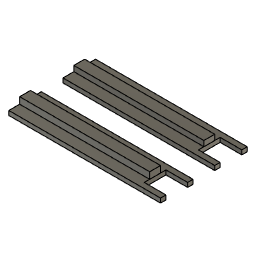
Abdeckung Profielschiene oben (Autodesk Fusion 360 design; units mm, degrees)
Autodesk Fusion 360 part; units mm, degrees
sketch "Skizze1" plane through (0, 0, 0) normal (0, 0, 1) x (1, 0, 0)
  line L0 (0, 0) -> (280, 0)
  line L1 (280, 0) -> (280, 30)
  line L2 (280, 30) -> (0, 30)
  line L3 (0, 30) -> (0, 0)
  dimension "d1" = 30
  dimension "d2" = 280
  constraint horizontal L0
  constraint vertical L1
  constraint horizontal L2
  constraint vertical L3
  constraint coincident L0.start L3.end
  measures "d1" distance of L0.start L2.end
  measures "d2" distance of L0.start L0.end
extrude "Extrusion1" add sketch "Skizze1" along normal blind 1 makes body 1
sketch "Skizze2" plane through (0, 0, 1) normal (0, 0, 1) x (-1, 0, 0)
  line L0 (0, -30) -> (0, 0)
  line L1 (0, 0) -> (-280, 0)
  line L2 (-280, 0) -> (-280, -30)
  line L3 (-280, -30) -> (0, -30)
  line L4 (0, -25) -> (-20, -25)
  line L5 (-20, -25) -> (-20, -5)
  line L6 (-20, -5) -> (0, -5)
  line L7 (0, -5) -> (0, -25)
  line L8 (-280, -25) -> (-260, -25)
  line L9 (-260, -25) -> (-260, -5)
  line L10 (-260, -5) -> (-280, -5)
  line L11 (-280, -5) -> (-280, -25)
  dimension "d5" = 20
  dimension "d6" = 20
  dimension "d7" = 5
  dimension "d8" = 5
  dimension "d9" = 20
  dimension "d10" = 20
  dimension "d11" = 5
  constraint horizontal L4
  constraint vertical L5
  constraint horizontal L6
  constraint vertical L7
  constraint coincident L0 L4.start
  constraint horizontal L8
  constraint vertical L9
  constraint horizontal L10
  constraint vertical L11
  constraint coincident L2 L8.start
  measures "d5" distance of L4.start L4.end
  measures "d6" distance of L4.start L6.end
  measures "d7" distance of L1 L6
  measures "d8" distance of L3 L4
  measures "d9" distance of L8.start L8.end
  measures "d10" distance of L8.start L10.end
  measures "d11" distance of L1 L10
extrude "Extrusion2" cut sketch "Skizze2" against normal blind 10 contours L0 L4 L5 L6 L7 | L2 L8 L9 L10 L11 bodies 1
sketch "Skizze3" plane through (0, 0, 1) normal (0, 0, 1) x (-1, 0, 0)
  line L0 (-260, -25) -> (-280, -25)
  line L1 (-280, -25) -> (-280, -30)
  line L2 (-280, -30) -> (0, -30)
  line L3 (0, -30) -> (0, -25)
  line L4 (0, -25) -> (-20, -25)
  line L5 (-20, -25) -> (-20, -5)
  line L6 (-20, -5) -> (0, -5)
  line L7 (0, -5) -> (0, 0)
  line L8 (0, 0) -> (-280, 0)
  line L9 (-280, 0) -> (-280, -5)
  line L10 (-280, -5) -> (-260, -5)
  line L11 (-260, -5) -> (-260, -25)
  line L12 (-259.9999, -20) -> (-20, -20)
  line L13 (-20, -20) -> (-20, -10)
  line L14 (-20, -10) -> (-259.9999, -10)
  line L15 (-259.9999, -10) -> (-259.9999, -20)
  dimension "d14" = 10
  dimension "d16" = 10
  constraint horizontal L12
  constraint vertical L13
  constraint horizontal L14
  constraint vertical L15
  measures "d14" distance of L8 L14
  measures "d16" distance of L2 L12
extrude "Extrusion3" add sketch "Skizze3" along normal blind 5 contours L5 L11 L12 L13 L14 L15 bodies 1
sketch "Skizze4" plane through (0, 0, 0) normal (0, 0, -1) x (1, 0, 0)
  line L0 (280, -25) -> (260, -25)
  line L1 (260, -25) -> (260, -5)
  line L2 (260, -5) -> (280, -5)
  line L3 (280, -5) -> (280, 0)
  line L4 (280, 0) -> (0, 0)
  line L5 (0, 0) -> (0, -5)
  line L6 (0, -5) -> (20, -5)
  line L7 (20, -5) -> (20, -25)
  line L8 (20, -25) -> (0, -25)
  line L9 (0, -25) -> (0, -30)
  line L10 (0, -30) -> (280, -30)
  line L11 (280, -30) -> (280, -25)
  line L12 (0, 0) -> (140, 0)
  line L13 (140, 0) -> (140, -30)
  line L14 (140, -30) -> (0, -30)
  line L15 (0, -30) -> (0, 0)
  dimension "d21" = 140
  constraint horizontal L12
  constraint vertical L13
  constraint horizontal L14
  constraint vertical L15
  constraint coincident L10 L13.end
  constraint coincident L4.end L5.start
  measures "d21" distance of L4.end L12.end
extrude "Extrusion4" cut sketch "Skizze4" against normal blind 15 contours L4 L5 L6 L7 L8 L9 L10 L12 L13 L14 L15 bodies 1
sketch "Skizze5" plane through (0, 0, 0) normal (0, 0, -1) x (1, 0, 0)
  line L0 (140, 0) -> (140, -30)
  line L1 (140, -30) -> (280, -30)
  line L2 (280, -30) -> (280, -25)
  line L3 (280, -25) -> (260, -25)
  line L4 (260, -25) -> (260, -5)
  line L5 (260, -5) -> (280, -5)
  line L6 (280, -5) -> (280, 0)
  line L7 (280, 0) -> (140, 0)
  line L8 (140, 10) -> (285, 10)
  line L9 (285, 10) -> (285, 5)
  line L10 (285, 5) -> (140, 5)
  line L11 (140, 5) -> (140, 10)
  line L12 (280, 45) -> (260, 45)
  line L13 (280, 50) -> (280, 45)
  line L14 (260, 25) -> (280, 25)
  line L15 (140, 50) -> (280, 50)
  line L16 (260, 45) -> (260, 25)
  line L17 (140, 20) -> (140, 50)
  line L18 (280, 20) -> (140, 20)
  line L19 (280, 25) -> (280, 20)
  constraint horizontal L8
  constraint vertical L9
  constraint horizontal L10
  constraint vertical L11
  constraint symmetric L0.start L8 L17.start
  constraint symmetric L0.end L8 L15.start
  constraint symmetric L1.end L8 L13.start
  constraint symmetric L2.end L8 L12.start
  constraint symmetric L3.end L8 L12.end
  constraint symmetric L4.end L8 L14.start
  constraint symmetric L5.end L8 L14.end
  constraint symmetric L6.end L8 L18.start
extrude "Extrusion5" add sketch "Skizze5" along normal blind 4 separate body contours L12 L13 L14 L15 L16 L17 L18 L19 makes body 2
extrude "Extrusion6" add 1 faces at (180, 18.3333, 0) along direction (0, 0, -1) blind 3 on bodies 1 bodies 1
sketch "Skizze6" plane through (0, 0, 6) normal (0, 0, 1) x (-1, 0, 0)
  line L0 (-140, -20) -> (-140, -10)
  line L1 (-140, -10) -> (-259.9999, -10)
  line L2 (-259.9999, -10) -> (-259.9999, -20)
  line L3 (-259.9999, -20) -> (-140, -20)
  line L4 (-280, 15) -> (-140, 15)
  line L5 (-140, 15) -> (-140, 9.9999)
  line L6 (-140, 9.9999) -> (-280, 9.9999)
  line L7 (-280, 9.9999) -> (-280, 15)
  line L8 (-140, 29.9999) -> (-259.9999, 29.9999)
  line L9 (-259.9999, 29.9999) -> (-259.9999, 39.9999)
  line L10 (-259.9999, 39.9999) -> (-140, 39.9999)
  line L11 (-140, 39.9999) -> (-140, 29.9999)
  constraint horizontal L4
  constraint vertical L5
  constraint horizontal L6
  constraint vertical L7
  constraint symmetric L0.start L6 L10.end
  constraint symmetric L0.end L6 L8.start
  constraint symmetric L1.end L6 L8.end
  constraint symmetric L2.end L6 L9.end
extrude "Extrusion7" add sketch "Skizze6" against normal blind 6 contours L8 L9 L10 L11 bodies 2
